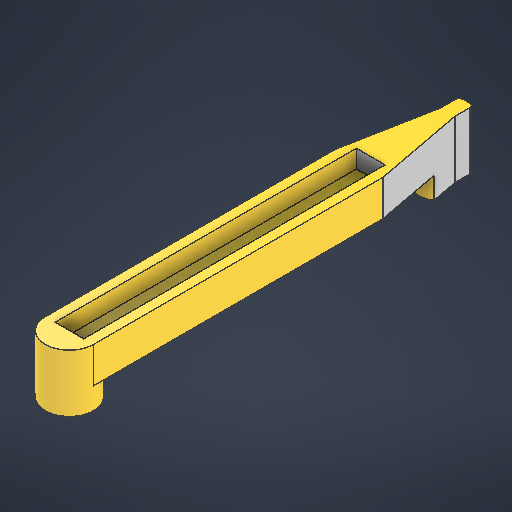
# Autodesk Inventor part: measuring_slider1
Saved by Autodesk Inventor 2026.1 (Build 301233000, 233)
## iProperties
Created: 2025-12-25
Part Number: measuring_slider1
Material: Generic
Document SubType Name: Modeling
Designer: emanuel
Density: 1 g/cm^3
Appearance: Default
Author: emanuel
Autodesk Inventor part; units mm, degrees
ref_plane "YZ Plane" through (0, 0, 0) normal (1, 0, 0) x (0, 1, 0)
ref_plane "XZ Plane" through (0, 0, 0) normal (0, 1, 0) x (-1, 0, 0)
ref_plane "XY Plane" through (0, 0, 0) normal (0, 0, 1) x (1, 0, 0)
sketch "Sketch1" plane through (0, 0, 0) normal (0, 1, 0) x (-1, 0, 0)
  circle A0 centre (0, 0) radius 3.35
  circle A1 centre (0, 0) radius 3.5
  line L0 (0, -3.5) -> (0, -48.5)
  line L1 (0, -48.5) -> (0, -52)
  circle A2 centre (0, -52) radius 3.35
  line L2 (3.35, 0) -> (-3.35, 0)
  line L3 (-3.35, 0) -> (-3.35, -52)
  line L4 (-3.35, -52) -> (3.35, -52)
  line L5 (3.35, -52) -> (3.35, 0)
  point P0 (3.35, -52)
  dimension "d0" = 6.7
  dimension "d1" = 7
  dimension "d4" = 6.7
  dimension "d2" = 45
  dimension "d3" = 3.5
  constraints: 12 end point, 3 coincident, 2 parallel, 2 vertical, 1 horizontal, 1 perpendicular, 1 vertical alignment, 8 other
  measures "d2" distance of L0.start L0.end
  measures "d3" distance of L0.end L1.end
extrude "Extrusion1" add sketch "Sketch1" along normal blind 2.5 contours L2 A0 | L5 A1 L3 A0 | A0 L2 | L5 A2 L1 L0 A1 | A1 L0 L1 A2 L3 | L4 L1 A2 | A2 L4 | A2 L1 L4 picked at (0, -3.3837)
sketch "Sketch2" plane through (0, 0, 0) normal (0, -1, 0) x (1, 0, 0)
  circle A0 centre (0, 0) radius 3.35
  arc A1 (-3.35, -52) -> (3.35, -52) centre (0, -52) ccw projected
  circle A2 centre (0, -52) radius 3.35
  point P0 (-3.35, -52)
  constraints: 2 coincident, 1 centre point, 3 other
extrude "Extrusion2" add sketch "Sketch2" along normal blind 3
sketch "Sketch3" plane through (0, 2.5, 0) normal (0, 1, 0) x (1, 0, 0)
  arc A0 (3.35, 52) -> (-3.35, 52) centre (0, 52) ccw projected
  line L0 (0, 52) -> (2, 52)
  line L1 (0, 0) -> (-2, 0)
  line L2 (-2, 0) -> (2, 0)
  line L3 (2, 0) -> (2, 52)
  line L4 (2, 52) -> (-2, 52)
  line L5 (-2, 52) -> (-2, 0)
  arc A1 (3.35, 52) -> (-3.35, 52) centre (0, 52) ccw
  line L6 (3.35, 0) -> (3.35, 52) projected
  line L7 (-3.35, 52) -> (3.35, 52)
  line L8 (3.35, 52) -> (3.35, 0)
  line L9 (3.35, 0) -> (-3.35, 0)
  line L10 (-3.35, 0) -> (-3.35, 52)
  arc A2 (-3.35, 0) -> (3.35, 0) centre (0, 0) ccw
  line L11 (-2, 52) -> (2, 52)
  line L12 (2, 52) -> (2, 42)
  line L13 (2, 42) -> (-2, 42)
  line L14 (-2, 42) -> (-2, 52)
  point P0 (-2, 42)
  dimension "d9" = 2
  dimension "d10" = 2
  dimension "d15" = 10
  constraints: 28 end point, 6 parallel, 5 horizontal, 5 point on circle, 3 perpendicular, 2 centre point, 2 coincident, 1 point on line
  measures "d9" distance of L0.start L0.end
  measures "d10" distance of L1.start L1.end
  measures "d15" distance of L11.end L12.end
extrude "Extrusion3" add sketch "Sketch3" along normal blind 2.5 contours L7 L0 L4 A0 | L6 L9 L3 L7 | L7 L5 L9 L10 | A2 L9 L1 L2 | L3 L13 L5 L4 L0
sketch "Sketch4" plane through (0, -3, 0) normal (0, -1, 0) x (1, 0, 0)
  circle A0 centre (0, 0) radius 3.5
  line L0 (2, -52) -> (-2, -52) projected
  circle A1 centre (0, -52) radius 3.5
  dimension "d13" = 7
  dimension "d14" = 7
  constraints: 2 centre point, 1 coincident, 1 midpoint
  measures "d13" diameter of A0
  measures "d14" diameter of A1
sketch "Sketch5" plane through (0, -3, -52) normal (0, -1, 0) x (1, 0, 0)
  arc A0 (-3.35, 0) -> (3.35, 0) centre (0, 0) ccw projected
  line L0 (0, -3.35) -> (0, 11.65)
  line L1 (0, 11.65) -> (3.35, 11.65)
  line L2 (3.35, 52) -> (3.35, 0) projected
  line L3 (0, 11.65) -> (-3.35, 11.65)
  line L4 (-3.35, 0) -> (-3.35, 52) projected
  line L5 (3.35, 11.65) -> (-3.35, 11.65)
  line L6 (-3.35, 11.65) -> (-3.35, 1.65)
  line L7 (3.35, 1.65) -> (3.35, 11.65)
  line L8 (3.35, 11.65) -> (-3.35, 11.65)
  line L9 (-3.35, 11.65) -> (-3.35, -3.35)
  line L10 (-3.35, -3.35) -> (3.35, -3.35)
  line L11 (3.35, -3.35) -> (3.35, 11.65)
  line L12 (0, -3.35) -> (2, -3.35)
  line L13 (2, -3.35) -> (-2, -3.35)
  line L14 (-2, -3.35) -> (-3.35, 11.65)
  line L15 (3.35, 11.65) -> (2, -3.35)
  line L16 (0, -3.35) -> (0, 6.65)
  line L17 (0, 6.65) -> (3.35, 6.65)
  line L18 (0, -3.35) -> (0.5, -3.35)
  line L19 (0.5, -3.35) -> (-0.5, -3.35)
  line L20 (0, 6.65) -> (-3.35, 6.65)
  line L21 (-0.5, -3.35) -> (-3.35, 6.65)
  line L22 (3.35, 6.65) -> (0.5, -3.35)
  line L23 (3.35, 11.65) -> (0.5, -3.35)
  line L24 (-3.35, 11.65) -> (-0.5, -3.35)
  line L25 (0, -3.35) -> (1, -3.35)
  line L26 (1, -3.35) -> (1, -0.7184)
  line L27 (1, -0.7184) -> (0, -0.7184)
  line L28 (0, -0.7184) -> (0, -3.35)
  arc A1 (3.35, 0) -> (-3.35, 0) centre (0, 0) ccw projected
  line L29 (0, -3.35) -> (-1.6865, -3.35)
  line L30 (0, 2.8945) -> (0, -3.35)
  line L31 (0, -3.35) -> (-1, -3.35)
  line L32 (-1, -3.35) -> (-1, -0.7184)
  line L33 (-1, -0.7184) -> (0, -0.7184)
  line L34 (0, -0.7184) -> (0, -3.35)
  point P0 (0, 52)
  point P1 (-2.064, -2.6386)
  point P2 (2.064, -2.6386)
  point P3 (-0.5112, -3.3108)
  point P4 (-2.6923, 4.3423)
  point P5 (2.6923, 4.3423)
  point P6 (0.5112, -3.3108)
  point P7 (-0.5073, -3.3114)
  point P8 (0.5073, -3.3114)
  point P9 (-1.6865, 2.8945)
  point P10 (1, -3.1973)
  point P11 (0, -3.35)
  point P12 (0, 11.65)
  point P13 (0, 11.65)
  point P14 (-1, -3.1973)
  dimension "d16" = 15
  dimension "d19" = 2
  dimension "d20" = 4
  dimension "d21" = 10
  dimension "d22" = 0.5
  dimension "d23" = 1
  dimension "d24" = 1
  constraints: 66 end point, 13 point on line, 7 parallel, 7 perpendicular, 5 horizontal, 1 point on circle, 1 vertical, 2 other
  measures "d16" distance of L0.start L0.end
  measures "d19" distance of L0.start L12.end
  measures "d20" distance of L12.end L13.end
  measures "d21" distance of L0.start L16.end
  measures "d22" distance of L0.start L18.end
  measures "d23" distance of L18.end L19.end
  measures "d24" distance between parallel lines of L0 L26
extrude "Extrusion4" cut sketch "Sketch5" against normal blind 10 contours A1 L14 A0 | L4 L21 L14 A1 | L14 A1 L21 L32 A0 | A0 L32 L10 L14 | L14 L21 A1 | A0 L21 L10 L32 | L4 L14 L20 | L20 L14 L21 | L14 L20 L24 A1 L21 | A1 L24 L32 L21 | L24 L20 L14 | L2 L17 L15 | L15 L17 L23 | A1 L22 L26 L23 | L23 L17 L15 L22 A1 | L26 L22 A1 L15 A0 | L22 L15 L17 | L2 A1 L15 L22 | L22 L15 A1 | L15 A1 A0
fillet "Fillet1" radius 0.5 2 edges at (1, 1, -55.1973) (-1, 1, -55.1973)
body "Solid1"
